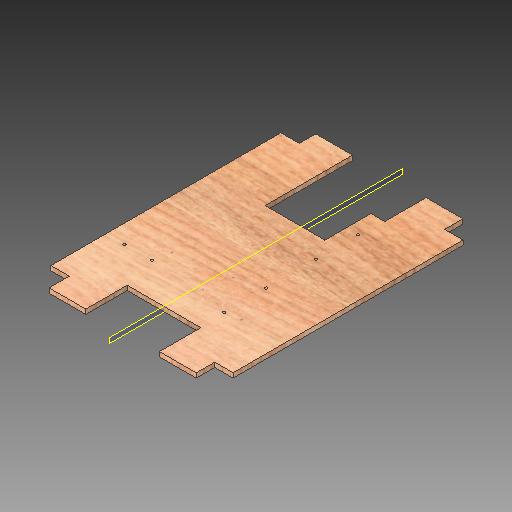
# Autodesk Inventor part: etage-bras
Saved by Autodesk Inventor 2019 (Build 230136000, 136)
## iProperties
Created: 2018-04-01
Part Number: etage-bras
Material: Générique
Document SubType Name: Modeling
Designer: franc
Density: 1 g/cm^3
Appearance: Par défaut
Mass: 72.5 g
Surface Area: 324 cm^2
Volume: 72.5 cm^3
Author: franc
Autodesk Inventor part; units mm, degrees
ref_plane "YZ Plane" through (0, 0, 0) normal (1, 0, 0) x (0, 1, 0)
ref_plane "XZ Plane" through (0, 0, 0) normal (0, 1, 0) x (-1, 0, 0)
ref_plane "XY Plane" through (0, 0, 0) normal (0, 0, 1) x (1, 0, 0)
sketch "Esquisse1" plane through (0, 0, 0) normal (0, 1, 0) x (-1, 0, 0)
  line L0 (57.703, 92.8408) -> (-102.297, 92.8408)
  line L1 (-102.297, -197.1592) -> (57.703, -197.1592)
  line L2 (-102.297, 72.7532) -> (-122.297, 72.7532)
  line L3 (-122.297, 72.7532) -> (-122.297, -177.2468)
  line L4 (-122.297, -177.2468) -> (-102.297, -177.2468)
  line L5 (-102.297, 70.8056) -> (-102.297, 72.7532)
  line L6 (57.703, 70.8056) -> (77.703, 70.8056)
  line L7 (77.703, 70.8056) -> (77.703, -179.1944)
  line L8 (77.703, -179.1944) -> (57.703, -179.1944)
  line L9 (57.703, -179.1944) -> (57.703, -177.2468)
  line L10 (57.703, -197.1592) -> (57.703, -179.1944)
  line L11 (57.703, 70.8056) -> (57.703, 92.8408)
  line L12 (-102.297, 92.8408) -> (-102.297, 72.7532)
  line L13 (-102.297, -177.2468) -> (-102.297, -197.1592)
  point P0 (0, 0)
  dimension "d0" = 290
  dimension "d1" = 160
  dimension "d17" = 20
  dimension "d18" = 250
  dimension "d19" = 20
  dimension "d20" = 250
  constraints: 28 end point, 9 parallel, 4 perpendicular, 3 horizontal, 2 point on line
  measures "d0" distance of L1.end L0.start
  measures "d1" distance of L0.start L0.end
  measures "d17" distance of L2.start L2.end
  measures "d18" distance of L2.end L3.end
  measures "d19" distance of L6.start L6.end
  measures "d20" distance of L6.end L7.end
extrude "Extrusion1" add sketch "Esquisse1" along normal blind 5
ref_plane "Plan de construction1" through (22.297, 0, -197.1592) normal (-1, 0, 0) x (0, 0, 1)
sketch "Sketch2" plane through (0, 5, 0) normal (0, 1, 0) x (1, 0, 0)
  circle A0 centre (60.447, -20.6408) radius 1.5001 projected
  circle A1 centre (60.447, 24.9592) radius 1.5 projected
  circle A2 centre (60.447, 124.9592) radius 1.5 projected
  circle A3 centre (60.447, 79.3592) radius 1.5 projected
  point P0 (0, 0)
extrude "Extrusion2" cut sketch "Sketch2" against normal through all
sketch "Sketch5" plane through (0, 5, 0) normal (0, 1, 0) x (1, 0, 0)
  line L0 (-17.703, -92.8408) -> (62.297, -92.8408)
  line L1 (62.297, -92.8408) -> (62.297, -47.8408)
  line L2 (62.297, -47.8408) -> (-17.703, -47.8408)
  line L3 (-17.703, -47.8408) -> (-17.703, -92.8408)
  line L4 (-57.703, -92.8408) -> (102.297, -92.8408) projected
  line L5 (-57.703, 197.1592) -> (-57.703, -92.8408) projected
  line L6 (102.297, -92.8408) -> (102.297, 197.1592) projected
  line L7 (102.297, 197.1592) -> (-57.703, 197.1592) projected
  line L8 (-17.703, 197.1592) -> (62.297, 197.1592)
  line L9 (62.297, 197.1592) -> (62.297, 152.1592)
  line L10 (62.297, 152.1592) -> (-17.703, 152.1592)
  line L11 (-17.703, 152.1592) -> (-17.703, 197.1592)
  line L12 (47.297, 152.1592) -> (-17.703, 152.1592)
  line L13 (-17.703, 152.1592) -> (-17.703, 102.1592)
  line L14 (-17.703, 102.1592) -> (47.297, 102.1592)
  line L15 (47.297, 102.1592) -> (47.297, 152.1592)
  point P0 (0, 0)
  dimension "d6" = 0
  dimension "d7" = 45
  dimension "d8" = 40
  dimension "d9" = 40
  dimension "d10" = 40
  dimension "d11" = 40
  dimension "d12" = 45
  dimension "d15" = 65
  dimension "d16" = 50
  constraints: 24 end point, 6 parallel, 3 horizontal, 3 perpendicular, 2 point on line
  measures "d6" distance between parallel lines of L4 L0
  measures "d7" distance between parallel lines of L2 L4
  measures "d8" distance between parallel lines of L5 L3
  measures "d9" distance between parallel lines of L6 L1
  measures "d10" distance between parallel lines of L5 L11
  measures "d11" distance between parallel lines of L6 L9
  measures "d12" distance of L8.end L9.end
  measures "d15" distance of L13.end L14.end
  measures "d16" distance of L14.end L12.start
extrude "Extrusion3" cut sketch "Sketch5" against normal through all contours L3 L2 L1 L0 | L7 L9 L10 L11 | L10 L15 L14 L13
sketch "Sketch6" plane through (0, 5, 0) normal (0, 1, 0) x (1, 0, 0)
  spline S0 degree 3 poles (-57.703, -9.3408) (-57.5164, -9.3408) (-57.3163, -9.3777) (-56.9466, -9.5301) (-56.7768, -9.6456) (-56.51, -9.9124) (-56.3945, -10.0805) (-56.241, -10.4501) (-56.203, -10.6516) (-56.203, -11.03) (-56.241, -11.2314) (-56.3945, -11.601) (-56.51, -11.7692) (-56.7768, -12.0359) (-56.9466, -12.1514) (-57.3163, -12.3038) (-57.5164, -12.3408) (-57.8926, -12.3408) (-58.0946, -12.3027) (-58.4667, -12.1475) (-58.6367, -12.0303) (-58.9007, -11.7625) (-59.0142, -11.5958) (-59.1654, -11.2291) (-59.203, -11.029) (-59.203, -10.6526) (-59.1654, -10.4525) (-59.0142, -10.0858) (-58.9007, -9.9191) (-58.6367, -9.6513) (-58.4667, -9.5341) (-58.0946, -9.3788) (-57.8926, -9.3408) (-57.703, -9.3408) knots 0 0 0 0 0.057709 0.057709 0.115418 0.115418 0.172176 0.172176 0.228935 0.228935 0.285694 0.285694 0.342453 0.342453 0.400161 0.400161 0.45787 0.45787 0.516493 0.516493 0.575116 0.575116 0.631571 0.631571 0.688026 0.688026 0.744481 0.744481 0.800936 0.800936 0.859558 0.859558 0.918181 0.918181 0.918181 0.918181 projected
  spline S1 degree 3 poles (-27.703, -9.3408) (-27.5152, -9.3408) (-27.314, -9.3782) (-26.9424, -9.5324) (-26.772, -9.6492) (-26.5065, -9.9173) (-26.3923, -10.0847) (-26.2405, -10.4525) (-26.203, -10.6528) (-26.203, -11.0288) (-26.2405, -11.229) (-26.3923, -11.5968) (-26.5065, -11.7643) (-26.772, -12.0324) (-26.9424, -12.1492) (-27.314, -12.3034) (-27.5152, -12.3408) (-27.8908, -12.3408) (-28.0911, -12.3034) (-28.4604, -12.1508) (-28.6295, -12.0356) (-28.8953, -11.7698) (-29.0108, -11.6022) (-29.1647, -11.2327) (-29.203, -11.0308) (-29.203, -10.6508) (-29.1647, -10.4489) (-29.0108, -10.0794) (-28.8953, -9.9118) (-28.6295, -9.646) (-28.4604, -9.5307) (-28.0911, -9.3781) (-27.8908, -9.3408) (-27.703, -9.3408) knots 0 0 0 0 0.058071 0.058071 0.116142 0.116142 0.172538 0.172538 0.228935 0.228935 0.285331 0.285331 0.341727 0.341727 0.399798 0.399798 0.457869 0.457869 0.515944 0.515944 0.574019 0.574019 0.631023 0.631023 0.688027 0.688027 0.74503 0.74503 0.802034 0.802034 0.860109 0.860109 0.918184 0.918184 0.918184 0.918184 projected
  point P0 (0, 0)
  point P1 (-57.703, -9.3408)
  point P2 (-27.703, -9.3408)
extrude "Extrusion4" cut sketch "Sketch6" against normal through all
